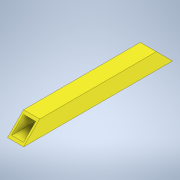
# Autodesk Inventor part: 9_250-inchAluminumTubingWith45DegreeCuts
Saved by Autodesk Inventor 2020.2 (Build 242310000, 310)
## iProperties
Created: 2020-01-17
Part Number: 9_250-inchAluminumTubingWith45DegreeCuts
Material: Aluminum 6061
Document SubType Name: Modeling
Designer: robst
Density: 2.7 g/cm^3
Appearance: Canary
Author: robst
Autodesk Inventor part; units mm, degrees
ref_plane "YZ Plane" through (0, 0, 0) normal (1, 0, 0) x (0, 1, 0)
ref_plane "XZ Plane" through (0, 0, 0) normal (0, 1, 0) x (-1, 0, 0)
ref_plane "XY Plane" through (0, 0, 0) normal (0, 0, 1) x (1, 0, 0)
sketch "Sketch1" plane through (0, 0, 0) normal (0, 0, 1) x (1, 0, 0)
  line L0 (-12.7, -12.7) -> (12.7, -12.7)
  line L1 (12.7, -12.7) -> (12.7, 12.7)
  line L2 (12.7, 12.7) -> (-12.7, 12.7)
  line L3 (-12.7, 12.7) -> (-12.7, -12.7)
  line L4 (-12.7, -12.7) -> (12.7, 12.7) construction
  line L5 (12.7, -12.7) -> (-12.7, 12.7) construction
  line L6 (-9.525, -9.525) -> (9.525, -9.525)
  line L7 (9.525, -9.525) -> (9.525, 9.525)
  line L8 (9.525, 9.525) -> (-9.525, 9.525)
  line L9 (-9.525, 9.525) -> (-9.525, -9.525)
  line L10 (-9.525, -9.525) -> (9.525, 9.525) construction
  line L11 (9.525, -9.525) -> (-9.525, 9.525) construction
  point P0 (0, 0)
  dimension "d0" = 25.4
  dimension "d1" = 25.4
  dimension "d2" = 3.175
  dimension "d3" = 3.175
  constraints: 24 end point, 4 midpoint, 4 parallel, 2 horizontal, 2 perpendicular
  measures "d0" distance of L0.start L0.end
  measures "d1" distance of L1.end L0.end
  measures "d2" distance between parallel lines of L6 L0
  measures "d3" distance between parallel lines of L3 L9
extrude "Extrusion1" add sketch "Sketch1" along normal mid plane 234.95
sketch "Sketch2" plane through (12.7, -12.7, 117.475) normal (1, 0, 0) x (0, 0, -1)
  line L0 (0, 0) -> (0, 25.4) projected
  line L1 (0, 0) -> (25.4, 25.4)
  line L2 (0, 25.4) -> (234.95, 25.4) projected
  line L3 (0, 25.4) -> (0, 0)
  line L4 (234.95, 0) -> (0, 0) projected
  line L5 (234.95, 0) -> (234.95, 25.4) projected
  line L6 (234.95, 0) -> (209.55, 25.4)
  line L7 (234.95, 25.4) -> (234.95, 0)
  point P0 (117.475, 12.7)
  dimension "d7" = 45
  dimension "d8" = 45
  constraints: 8 end point, 2 point on line, 1 perpendicular, 1 vertical
  measures "d7" angle of L1 L4
  measures "d8" angle of L6 L4
extrude "Extrusion2" cut sketch "Sketch2" against normal through all contours L0 L2 L1 | L6 L2 L5
body "Solid1"
